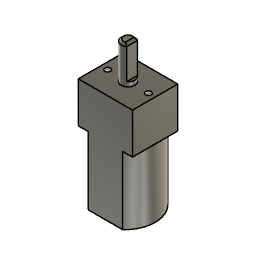
Gripper-3dita v34 (Autodesk Fusion 360 archive; units mm, degrees)
design "motore N20 A2.60RPM"
Autodesk Fusion 360 part; units mm, degrees
sketch "Schizzo1" plane through (0, 0, 0) normal (0, 0, 1) x (1, 0, 0)
  line L0 (-14.6061, 11.2687) -> (-2.6061, 11.2687) construction
  line L1 (-2.6061, 11.2687) -> (-2.6061, 1.2687)
  line L2 (-2.6061, 1.2687) -> (-14.6061, 1.2687) construction
  line L3 (-14.6061, 1.2687) -> (-14.6061, 11.2687)
  line L4 (-12.4061, 11.2687) -> (-4.8061, 11.2687)
  line L5 (-12.4061, 1.2687) -> (-4.8061, 1.2687)
  arc A0 (-12.4061, 11.2687) -> (-12.4061, 1.2687) centre (-7.8242, 6.2687) ccw
  arc A1 (-4.8061, 1.2687) -> (-4.8061, 11.2687) centre (-9.3879, 6.2687) ccw
  line L6 (-14.6061, 11.2687) -> (-2.6061, 1.2687)
  line L7 (-2.6061, 11.2687) -> (-14.6061, 1.2687)
  line L8 (-22.6061, 6.2687) -> (5.3939, 6.2687)
  dimension "d1" = 10
  dimension "d2" = 12
  dimension "d5" = 7.6
  dimension "d6" = 7.6
  constraint horizontal L0
  constraint vertical L1
  constraint horizontal L2
  constraint vertical L3
  constraint coincident L0 L4.start
  constraint parallel L0 L4
  constraint coincident L2 L5.start
  constraint parallel L2 L5
  constraint equal A0 A1
  constraint tangent L3 A0
  constraint tangent L1 A1
  constraint horizontal L8
  constraint midpoint L7 L8
  constraint coincident A1.centre L8
  measures "d1" distance of L0.start L2.end
  measures "d2" distance of L0.start L0.end
  measures "d5" distance of L4.start L4.end
  measures "d6" distance of L5.start L5.end
extrude "Estrusione1" add sketch "Schizzo1" along normal blind 15 contours A1 L7 L8 | A1 L6 L8 | L4 A0 A1 L6 L7 | L5 A0 A1 L6 L7 | A0 L6 L8 | A0 L7 L8
sketch "Schizzo2" plane through (0, 0, 15) normal (0, 0, 1) x (-1, 0, 0)
  arc A0 (12.4061, -11.2687) -> (12.4061, -1.2687) centre (7.8242, -6.2687) ccw
  line L0 (12.4061, -1.2687) -> (4.8061, -1.2687)
  arc A1 (4.8061, -1.2687) -> (4.8061, -11.2687) centre (9.3879, -6.2687) ccw
  line L1 (4.8061, -11.2687) -> (12.4061, -11.2687)
  line L2 (14.6061, -11.2687) -> (2.6061, -11.2687)
  line L3 (2.6061, -11.2687) -> (2.6061, -1.2687)
  line L4 (2.6061, -1.2687) -> (14.6061, -1.2687)
  line L5 (14.6061, -1.2687) -> (14.6061, -11.2687)
  constraint horizontal L2
  constraint vertical L3
  constraint horizontal L4
  constraint vertical L5
  constraint collinear L0 L4
  constraint collinear L1 L2
  constraint tangent A1 L3
  constraint tangent A0 L5
extrude "Estrusione2" add sketch "Schizzo2" along normal blind 9
sketch "Schizzo3" plane through (0, 0, 24) normal (0, 0, 1) x (-1, 0, 0)
  line L0 (14.6061, -1.2687) -> (2.6061, -1.2687)
  line L1 (2.6061, -1.2687) -> (2.6061, -11.2687)
  line L2 (2.6061, -11.2687) -> (14.6061, -11.2687)
  line L3 (14.6061, -11.2687) -> (14.6061, -1.2687)
  line L4 (8.6061, -1.2687) -> (8.6061, -11.2687)
  circle A0 centre (8.6061, -6.2687) radius 1.5
  dimension "d9" = 3
  constraint midpoint L0 L4.start
  constraint midpoint L2 L4.end
  constraint midpoint L4 A0.centre
  measures "d9" diameter of A0
extrude "Estrusione3" add sketch "Schizzo3" along normal blind 1 contours L4 A0 | L4 A0
sketch "Schizzo4" plane through (0, 0, 25) normal (0, 0, 1) x (-1, 0, 0)
  circle A0 centre (8.6061, -6.2687) radius 1.5
  line L0 (7.7061, -7.4687) -> (7.7061, -3.5)
  line L1 (7.7061, -3.5) -> (10.1061, -3.5)
  line L2 (10.1061, -3.5) -> (10.1061, -6.2687)
  arc A1 (7.7061, -7.4687) -> (7.7061, -5.0687) centre (8.6061, -6.2687) ccw
  dimension "d12" = 3
  dimension "d13" = 2.4
  constraint concentric A0 A1
  constraint vertical L0
  constraint horizontal L1
  constraint vertical L2
  constraint tangent L2 A1
  constraint coincident A0 L2.end
  constraint coincident A0 L0.start
  constraint coincident L0 A1.end
  measures "d12" diameter of A1
  measures "d13" distance of L0.end L1.end
extrude "Estrusione4" add sketch "Schizzo4" along normal blind 7.2 contours A0 L0 A1
chamfer "Smusso1" distance 0.5 angle 45 1 faces at (-8.4844, 6.1233, 32.2)
sketch "Schizzo5" plane through (0, 0, 0) normal (0, 0, -1) x (1, 0, 0)
  arc A0 (-12.4061, -1.2687) -> (-12.4061, -11.2687) centre (-7.8242, -6.2687) ccw
  line L0 (-12.4061, -11.2687) -> (-4.8061, -11.2687)
  arc A1 (-4.8061, -11.2687) -> (-4.8061, -1.2687) centre (-9.3879, -6.2687) ccw
  line L1 (-4.8061, -1.2687) -> (-12.4061, -1.2687)
  circle A2 centre (-12.3093, -6.2383) radius 1.5561
  circle A3 centre (-5.3753, -6.1228) radius 1.5561
  constraint equal A2 A3
extrude "Estrusione5" add sketch "Schizzo5" along normal blind 2.039 contours A2 | A3
fillet "Raccordo1" radius 1.5 2 faces at (-12.7379, 6.5305, -2.039) (-4.8514, 6.3478, -2.039)
sketch "Schizzo6" plane through (0, 0, 24) normal (0, 0, 1) x (-1, 0, 0)
  circle A0 centre (8.6061, -6.2687) radius 1.5
  line L0 (14.6061, -1.2687) -> (2.6061, -1.2687)
  line L1 (2.6061, -1.2687) -> (2.6061, -11.2687)
  line L2 (2.6061, -11.2687) -> (14.6061, -11.2687)
  line L3 (14.6061, -11.2687) -> (14.6061, -1.2687)
  line L4 (13.1061, -6.2687) -> (4.1061, -6.2687)
  point P0 (13.1061, -6.2687)
  point P1 (4.1061, -6.2687)
  dimension "d21" = 9
  constraint perpendicular L3 L4
  constraint midpoint A0.centre L4
  constraint coincident P0 L4.start
  constraint coincident P1 L4.end
  measures "d21" distance of P0 P1
hole "Foratura1" at (-13.1061, 6.2687, 24) at (-4.1061, 6.2687, 24) direction (0, 0, -1) diameter 1.271 depth 6 tip angle 118
thread "Filettatura1" "ISO Metric profile 1.6 M1.6x0.35 6H" thread offset 0 thread depth 7.4

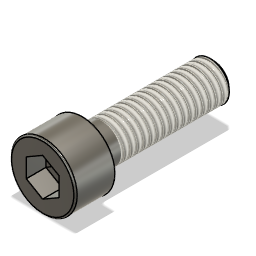
design "Vite a testa incassata JIS B 1176 - M6 x 1 x 20 Acciaio 4.6 Radente"
description: Vite a testa incassata JIS B 1176 - M6 x 1 x 20
part number: JIS B 1176 - M6 x 1 x 20 Acciaio 4.6 Radente
Autodesk Fusion 360 part; units mm, degrees
sketch "Sketch1" plane through (0, 0, 0) normal (0, 1, 0) x (1, 0, 0)
  line L0 (-3, 0) -> (-3, 20)
  line L1 (-3, 20) -> (0, 20)
  line L2 (0, 20) -> (0, -6)
  line L3 (-3, 0) -> (-5, 0)
  line L4 (-5, 0) -> (-5, -6)
  line L5 (-5, -6) -> (0, -6)
  dimension "d9" = 6
  dimension "d66" = 10
  dimension "d108" = 20
  dimension "d109" = 6
  constraint perpendicular L0 L1
  constraint collinear origin L1.end L2.end
  constraint perpendicular L0 L3
  constraint coincident origin L3
  constraint vertical L0
  constraint vertical L2
  constraint parallel L2 L4
  constraint coincident L2 L5.end
  constraint perpendicular L2 L5
  measures "d108" distance of origin L1
  measures "d109" distance of L3.end L5
revolve "Revolve1" add sketch "Sketch1" angle 360 about axis through (0, 0, -20) along (0, 0, 1)
ref_plane "WorkPlane1" through (0, 0, 6) normal (0, 0, 1) x (1, 0, 0)
sketch "Sketch6" plane through (0, 0, 6) normal (0, 0, 1) x (1, 0, 0)
  line L0 (-2.5, 0) -> (2.5, 0) construction
  line L1 (0, 0) -> (-2.5, 1.4434)
  line L2 (-2.5, -1.4434) -> (-2.5, 1.4434)
  line L3 (-2.5, -1.4434) -> (0, 0)
  dimension "d97" = 150
  dimension "d110" = 5
  constraint horizontal L0
  constraint midpoint L1.start L0
  constraint coincident L1.start L3.end
  constraint perpendicular L0 L2
  constraint midpoint L0.start L2
  constraint coincident L1.end L2.end
  measures "d97" angle of L0 L1
  measures "d110" distance of L0.end L2
extrude "Extrude1" cut sketch "Sketch6" against normal blind 3
pattern_circular "C-Pattern1" count 6 over 360 about axis through (0, 0, 1.75) along (0, 0, 1) of "Extrude1"
extrude "Extrude2" cut 1 faces at (0.8333, -0.4811, 3) along direction (0, 0, -1) blind 3 draft -85
thread "Thread2" "ISO Metric profile 6.0 M6x1 6g" major diameter 5.884 minor diameter 4.7435 pitch 1 angle 60 resizes the face on face at (-2.9851, 0.2987, -13.3333) from (0, 0, -3) to (0, 0, -20)
sketch "Sketch7" plane through (0, 0, 0) normal (0, 1, 0) x (1, 0, 0)
  line L0 (-3.06, 20) -> (-3.06, 19.3865)
  line L1 (-3.06, 19.3865) -> (-2.3865, 20)
  line L2 (0, 20) -> (0, -6)
  line L3 (-3.06, 20) -> (0, 20)
  dimension "d111" = 2.3866
  dimension "d112" = 3.06
  dimension "d113" = 0.6135
  constraint coincident L2.start L3.end
  constraint perpendicular L0 L3
  constraint coincident L1.end L3
  constraint perpendicular L2 L3
  measures "d111" distance of L1.end L2
  measures "d112" distance of L0 L2.start
  measures "d113" distance of L0.end L3
revolve "Revolve3" cut sketch "Sketch7" angle 360 about axis through (0, 0, 1.75) along (0, 0, 1)
fillet "Fillet5" radius 0.25 1 edges at (-4.6616, 1.8081, 6)
fillet "Fillet7" radius 0.6 1 edges at (2.7429, -1.0639, 0)
equation "d9 = adsk_nomdia"
equation "adsk_nomlen = 20.00 mm"
equation "adsk_headh = 6.00 mm"
equation "adsk_headdia = 10.00 mm"
equation "adsk_nomdia = 6.00 mm"
equation "adsk_philwidth = 5.00 mm"
equation "d31 = -adsk_phildepth"
equation "adsk_phildepth = 3.00 mm"
equation "d66 = adsk_headdia"
equation "d71 = adsk_headh"
equation "d76 = -adsk_phildepth"
equation "adsk_thrlen = 17.00 mm"
equation "d84 = adsk_thrlen"
equation "adsk_startlen = 0.61345 mm"
equation "adsk_endpointdia = 4.7731 mm"
equation "adsk_headtoprad = 0.25 mm"
equation "d102 = adsk_headtoprad"
equation "adsk_midfillet = 0.60 mm"
equation "d107 = adsk_midfillet"
equation "d108 = adsk_nomlen"
equation "d109 = adsk_headh"
equation "d110 = adsk_philwidth"
equation "d111 = adsk_endpointdia / 2"
equation "d112 = adsk_nomdia * 0.51"
equation "d113 = adsk_startlen"

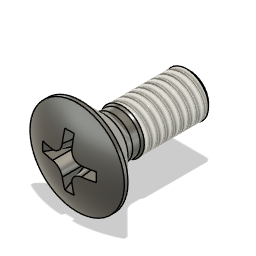
design "Vite a testa rialzata svasata UNI EN ISO 7047 - M4 x 10 - H Acciaio 4.6 Radente"
description: Vite a testa rialzata svasata UNI EN ISO 7047 - M4 x 10 - H
part number: UNI EN ISO 7047 - M4x10 - H Acciaio 4.6 Radente
Autodesk Fusion 360 part; units mm, degrees
sketch "Sketch1" plane through (0, 0, 0) normal (0, 1, 0) x (1, 0, 0)
  line L0 (-4.2, -4.525) -> (-4.2, -4.2)
  line L1 (-4.2, -4.2) -> (-1.825, -1.825)
  line L2 (-2, 5.475) -> (0, 5.475)
  line L3 (0, 5.475) -> (0, -5.525)
  arc A0 (-4.2, -4.525) -> (0, -5.525) centre (0, 3.795) ccw
  line L4 (-1.825, -1.825) -> (-1.825, -0.7281)
  line L5 (-2, -0.425) -> (-2, 5.475)
  line L6 (-2, -0.425) -> (-1.825, -0.7281)
  dimension "d9" = 4
  dimension "d11" = 8.4
  dimension "d68" = 10
  dimension "d90" = 2.7
  dimension "d91" = 1
  dimension "d93" = 3.65
  dimension "d135" = 5.9
  dimension "d157" = 45
  dimension "d160" = 30
  constraint vertical L0
  constraint vertical L3
  constraint coincident L3.end A0
  constraint coincident L3 A0.centre
  constraint vertical L4
  constraint parallel L4 L5
  constraint horizontal L2
  constraint coincident origin L3
  constraint coincident origin L1
  measures "d68" vertical distance of L0.start L2.start
  measures "d90" vertical distance of L0.start L1.end
  measures "d91" vertical distance of L3.end L0.start
  measures "d135" distance of L2 L5.start
  measures "d157" angle of L1 L3
  measures "d160" angle of L5 L6
revolve "Revolve1" add sketch "Sketch1" angle 360 about axis through (0, 0, -5.475) along (0, 0, 1) makes body 1
ref_plane "WorkPlane1" through (0, 0, 5.525) normal (0, 0, 1) x (1, 0, 0)
sketch "Sketch2" plane through (0, 0, 5.525) normal (0, 0, 1) x (1, 0, 0)
  line L0 (-0.4333, 2.6) -> (-0.4333, 0.4333)
  line L1 (-0.4333, 0.4333) -> (-2.6, 0.4333)
  line L2 (0, 0) -> (0, 2.6) construction
  line L3 (-0.4333, 2.6) -> (0.4333, 2.6)
  line L4 (-2.6, 0.4333) -> (-2.6, -0.4333)
  circle A0 centre (0, 0) radius 4.2
  line L5 (0, 0) -> (-4.2, 0) construction
  line L6 (2.6, 0.4333) -> (2.6, -0.4333)
  line L7 (0.4333, 0.4333) -> (2.6, 0.4333)
  line L8 (0.4333, 2.6) -> (0.4333, 0.4333)
  line L9 (-0.4333, -0.4333) -> (-2.6, -0.4333)
  line L10 (-0.4333, -2.6) -> (-0.4333, -0.4333)
  line L11 (-0.4333, -2.6) -> (0.4333, -2.6)
  line L12 (0.4333, -2.6) -> (0.4333, -0.4333)
  line L13 (0.4333, -0.4333) -> (2.6, -0.4333)
  dimension "d22" = 0.8667
  dimension "d161" = 5.2
  constraint perpendicular L0 L1
  constraint equal L3 L4
  constraint equal L0 L1
  constraint horizontal L0.start L2.end
  constraint vertical L2
  constraint coincident L2.start A0.centre
  constraint perpendicular L4 L5
  constraint coincident A0 L5.end
  constraint horizontal L5
  constraint vertical L0
  constraint symmetric L0.start L2 L3.end
  constraint symmetric L0.end L2 L7.start
  constraint symmetric L1.end L2 L6.start
  constraint symmetric L2 L4.end L6.end
  constraint coincident L3.end L8.start
  constraint symmetric L0.start L5 L10.start
  constraint symmetric L0.end L5 L9.start
  constraint symmetric L1.end L5 L4.end
  constraint symmetric L3.end L5 L11.end
  constraint symmetric L5 L6.start L6.end
  constraint symmetric L5 L7.start L12.end
  constraint symmetric L5 L3.end L11.end
  constraint coincident L6.end L13.end
  measures "d22" horizontal distance of L0.start L3.end
  measures "d161" distance of L1.end L6.start
extrude "Extrude1" add sketch "Sketch2" against normal blind 3.2 draft -4 separate body contours L0 L1 L3 L4 L6 L7 L8 L9 L10 L11 L12 L13 makes body 2
draft "Draft1" angle -30 neutral plane through (0, 0, 5.525) pull (0, 0, 1) 4 faces at (-2.5254, 0.0699, 4.4583) (0.0699, 2.5254, 4.4583) (0.0699, -2.5254, 4.4583) (2.5254, 0.0699, 4.4583) on bodies 2
fillet "Fillet3" radius 0.8667 4 edges at (-0.3215, 0.3215, 3.925) (0.3215, 0.3215, 3.925) (0.3215, -0.3215, 3.925) (-0.3215, -0.3215, 3.925) on bodies 2
combine "Combine1" operation cut target body 1 tool bodies 2
fillet "Fillet7" radius 1 1 edges at (-1.7015, 0.6599, 1.825) on bodies 1
thread "Thread1" "ISO Metric profile 4.0 M4x0.7 6g" major diameter 3.908 minor diameter 3.111 pitch 0.7 angle 60 resizes the face on face at (-1.9975, 0.0997, -1.5417) on bodies 1
sketch "Sketch7" plane through (0, 0, 0) normal (0, 1, 0) x (1, 0, 0)
  line L0 (-1.69, 5.475) -> (-2.04, 5.475)
  line L1 (-2.04, 5.475) -> (-2.04, 5.125)
  line L2 (-2.04, 5.125) -> (-1.69, 5.475)
  point P0 (0, 5.475)
  dimension "d152" = 45
  dimension "d154" = 0.35
  dimension "d155" = 2.04
  constraint horizontal L0
  constraint perpendicular L0 L1
  constraint coincident L0 P0
  measures "d152" angle of L1 L2
  measures "d154" distance of L0.end L1.end
  measures "d155" distance of L1 P0
revolve "Revolve3" cut sketch "Sketch7" angle 360 about axis through (0, 0, 1.75) along (0, 0, 1) bodies 1
equation "d9 = adsk_nomdia"
equation "d11 = adsk_headdia"
equation "d22 = adsk_philwidth"
equation "d31 = -adsk_phildepth"
equation "d59 = adsk_philwidth"
equation "d68 = adsk_nomlen"
equation "d71 = adsk_shnkdia * 0.5 / tan(adsk_headang * 0.5) + adsk_headh + adsk_ovalh"
equation "d90 = adsk_headh"
equation "d91 = adsk_ovalh"
equation "d93 = adsk_shnkdia"
equation "adsk_headang = 90.00 deg"
equation "adsk_nomlen = 10.00 mm"
equation "adsk_headh = 2.70 mm"
equation "adsk_headdia = 8.40 mm"
equation "adsk_nomdia = 4.00 mm"
equation "adsk_phildia = 5.20 mm"
equation "adsk_philwidth = adsk_phildia / 6"
equation "adsk_phildepth = 3.20 mm"
equation "adsk_ovalh = 1.00 mm"
equation "adsk_thrlen = 5.90 mm"
equation "adsk_shnkdia = adsk_nomdia - 0.5 * adsk_pitch1"
equation "d135 = adsk_thrlen"
equation "adsk_pitch1 = 0.70 mm"
equation "adsk_midfillet = 1.00 mm"
equation "d143 = adsk_midfillet"
equation "d150 = ( adsk_shnkdia * 0.5 ) * tan(90 deg - adsk_headang * 0.5) + adsk_headh"
equation "d154 = adsk_pitch1 * 0.5"
equation "d155 = adsk_nomdia * 0.51"
equation "d161 = adsk_phildia"

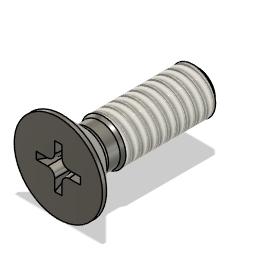
design "Vite a testa piatta svasata UNI EN ISO 7046-1 - M2 x 6 - H Acciaio 4.6 Radente"
description: Vite a testa piatta svasata UNI EN ISO 7046-1 - M2 x 6 - H
part number: UNI EN ISO 7046-1 - M2 x 6 - H Acciaio 4.6 Radente
Autodesk Fusion 360 part; units mm, degrees
sketch "Sketch1" plane through (0, 0, 0) normal (0, 1, 0) x (1, 0, 0)
  line L0 (0, -2.0773) -> (-1.9, -2.0773)
  line L1 (-1.9, -2.0773) -> (-1.9, -1.9)
  line L2 (-1.9, -1.9) -> (-0.8773, -0.8773)
  line L3 (-1, -0.0773) -> (-1, 3.9227)
  line L4 (-0.8773, -0.8773) -> (0, 0) construction
  line L5 (-1, 3.9227) -> (0, 3.9227)
  line L6 (0, 3.9227) -> (0, -2.0773)
  line L7 (-0.8773, -0.2898) -> (-0.8773, -0.8773)
  line L8 (-1, -0.0773) -> (-0.8773, -0.2898)
  dimension "d5" = 45
  dimension "d9" = 2
  dimension "d11" = 3.8
  dimension "d71" = 1.2
  dimension "d72" = 1.7546
  dimension "d89" = 4
  dimension "d101" = 30
  dimension "d115" = 6
  constraint perpendicular L0 L1
  constraint vertical L3
  constraint perpendicular L3 L5
  constraint collinear L2 L4
  constraint perpendicular L0 L6
  constraint collinear L4.end L0.start L5.end
  constraint coincident L4.end L6
  constraint coincident origin L4
  constraint horizontal L0
  constraint coincident L2.end L4.start
  constraint coincident L7 L8.end
  constraint coincident L7.start L8.end
  measures "d5" angle of L4 L6
  measures "d71" distance of L0 L2.end
  measures "d89" distance of L5 L3.start
  measures "d101" angle of L3 L8
  measures "d115" distance of L0.start L5
revolve "Revolve1" add sketch "Sketch1" angle 360 about axis through (0, 0, -3.9227) along (0, 0, 1) makes body 1
sketch "Sketch2" plane through (0, 0, 2.0773) normal (0, 0, 1) x (1, 0, 0)
  line L0 (-0.155, 0.155) -> (-0.95, 0.155)
  line L1 (-0.95, 0.155) -> (-0.95, -0.155)
  line L2 (-0.95, -0.155) -> (-0.155, -0.155)
  line L3 (0.155, -0.95) -> (0.155, -0.155)
  line L4 (-0.155, -0.95) -> (0.155, -0.95)
  line L5 (-0.155, -0.155) -> (-0.155, -0.95)
  line L6 (0.95, 0.155) -> (0.155, 0.155)
  line L7 (0.95, -0.155) -> (0.95, 0.155)
  line L8 (0.155, -0.155) -> (0.95, -0.155)
  line L9 (-0.155, 0.95) -> (-0.155, 0.155)
  line L10 (0.155, 0.95) -> (-0.155, 0.95)
  line L11 (0.155, 0.155) -> (0.155, 0.95)
  dimension "d111" = 360
  dimension "d116" = 0.31
  dimension "d117" = 1.9
  constraint horizontal L0
  constraint perpendicular L0 L1
  constraint horizontal L2
  constraint vertical L0.start L2.end
  constraint coincident L0.start L9.end
  measures "d116" distance of L0 L1.end
  measures "d117" distance of L4.start L10
extrude "Extrude1" add sketch "Sketch2" against normal blind 1.2 draft -4 separate body makes body 2
draft "Draft1" angle -30 neutral plane through (0, 0, 2.0773) pull (0, 0, 1) 4 faces at (0.922, 0.0237, 1.6773) (-0.0237, 0.922, 1.6773) (-0.922, -0.0237, 1.6773) (0.0237, -0.922, 1.6773) on bodies 2
fillet "Fillet3" radius 0.31 4 edges at (0.113, 0.113, 1.4773) (0.113, -0.113, 1.4773) (-0.113, -0.113, 1.4773) (-0.113, 0.113, 1.4773) on bodies 2
combine "Combine1" operation cut target body 1 tool bodies 2
thread "Thread1" "ISO Metric profile 2.0 M2x0.4 6g" major diameter 1.9335 minor diameter 1.478 pitch 0.4 angle 60 resizes the face on face at (-0.9988, 0.0498, -1.256) on bodies 1
fillet "Fillet5" radius 0.2 1 edges at (-0.8179, 0.3172, 0.8773) on bodies 1
sketch "Sketch6" plane through (0, 0, 0) normal (0, 1, 0) x (1, 0, 0)
  line L0 (-0.7546, 3.9227) -> (-1.02, 3.9227)
  line L1 (-1.02, 3.9227) -> (-1.02, 3.6773)
  line L2 (-1.02, 3.6773) -> (-0.7546, 3.9227)
  line L3 (-1, 3.9227) -> (0, 3.9227)
  line L4 (0, 0) -> (0, 3.9227) construction
  dimension "d102" = 1.02
  dimension "d118" = 0.7546
  dimension "d119" = 0.2454
  constraint horizontal L0
  constraint perpendicular L0 L1
  constraint coincident L0.start L3
  constraint coincident L4.start origin
  constraint coincident L3.end L4.end
  measures "d102" distance of L4.start L1
  measures "d118" distance of L0.start L4
  measures "d119" distance of L0 L1.end
revolve "Revolve3" cut sketch "Sketch6" angle 360 about axis through (0, 0, 1.75) along (0, 0, 1) bodies 1
equation "d5 = adsk_headang * 0.5"
equation "d9 = adsk_nomdia"
equation "d11 = adsk_headdia"
equation "adsk_nomlen = 6.00 mm"
equation "adsk_headh = 1.20 mm"
equation "adsk_headdia = 3.80 mm"
equation "adsk_nomdia = 2.00 mm"
equation "adsk_headang = 90.00 deg"
equation "adsk_phildia = 1.90 mm"
equation "d31 = -adsk_phildepth"
equation "adsk_philwidth = 0.31 mm"
equation "adsk_phildepth = 1.20 mm"
equation "d71 = adsk_headh"
equation "d72 = adsk_shnkdia"
equation "adsk_shnkdia = 1.75462 mm"
equation "d89 = adsk_thrlen"
equation "adsk_thrlen = 4.00 mm"
equation "adsk_pitch1 = 0.40 mm"
equation "adsk_startlen = 0.24538 mm"
equation "adsk_midfillet = adsk_nomdia * 0.1"
equation "d96 = adsk_midfillet"
equation "d99 = ( adsk_shnkdia / 2 ) * tan(90 deg - adsk_headang / 2) + adsk_headh"
equation "d102 = adsk_nomdia * 0.51"
equation "adsk_endpointdia = 1.50924 mm"
equation "d114 = adsk_philwidth"
equation "d115 = adsk_nomlen"
equation "d116 = adsk_philwidth"
equation "d117 = adsk_phildia"
equation "d118 = adsk_endpointdia / 2"
equation "d119 = adsk_startlen"

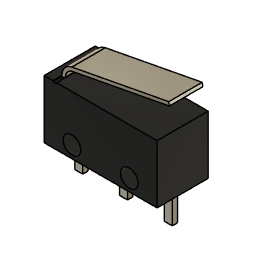
design "microswitch"
Autodesk Fusion 360 part; units mm, degrees
sketch "Schizzo1" plane through (0, 0, 0) normal (0, 1, 0) x (1, 0, 0)
  line L0 (0, 0) -> (12.8, 0)
  line L1 (12.8, 0) -> (12.8, -6.6)
  line L2 (12.8, -6.6) -> (0, -6.6)
  line L3 (0, -6.6) -> (0, 0)
  circle A0 centre (3.15, -1.35) radius 1
  circle A1 centre (9.65, -1.35) radius 1
  line L4 (0, -1.35) -> (3.15, -1.35) construction
  line L5 (3.15, -1.35) -> (9.65, -1.35) construction
  line L6 (9.65, -1.35) -> (12.8, -1.35) construction
  line L7 (1, -6.6) -> (1, -6.5)
  line L8 (1, -6.5) -> (1.4, -6.5)
  line L9 (1.4, -6.5) -> (1.4, -6.6)
  dimension "d1" = 6.6
  dimension "d2" = 12.8
  dimension "d3" = 2
  dimension "d4" = 2
  dimension "d5" = 6.5
  dimension "d6" = 5.25
  dimension "d7" = 1
  dimension "d8" = 0.1
  dimension "d9" = 0.4
  dimension "d28" = 6.6
  constraint horizontal L0
  constraint vertical L1
  constraint horizontal L2
  constraint vertical L3
  constraint coincident L0.start L3.end
  constraint coincident L3 L4.start
  constraint coincident A0.centre L4.end
  constraint perpendicular L3 L4
  constraint coincident A1.centre L5.end
  constraint coincident L1 L6.end
  constraint perpendicular L1 L6
  constraint horizontal L5
  constraint equal L4 L6
  constraint coincident L2 L7.start
  constraint perpendicular L2 L7
  constraint perpendicular L7 L8
  constraint coincident L2 L9.end
  constraint perpendicular L2 L9
  measures "d1" distance of L0.start L2.end
  measures "d2" distance of L0.start L0.end
  measures "d3" diameter of A0
  measures "d4" diameter of A1
  measures "d5" distance of A0.centre A1.centre
  measures "d6" distance of L2 L5
  measures "d7" distance of L3 L7
  measures "d8" distance of L7.start L7.end
  measures "d9" distance of L7.end L8.end
  measures "d28" distance of L0.end L1.end
extrude "Estrusione1" add sketch "Schizzo1" along normal mid plane 5.8 contours L0 L1 L2 L3 L7 L8 L9 makes body 1
sketch "Schizzo2" plane through (0, 0, 0) normal (0, 1, 0) x (1, 0, 0)
  arc A0 (1.4, -6.6275) -> (2.2125, -7.6097) centre (2.4, -6.6275) ccw
  line L0 (2.2125, -7.6097) -> (13.2, -9.7071)
  line L1 (0, -6.6) -> (0, 0)
  line L2 (0, 0) -> (12.8, 0)
  arc A1 (1, -6.6275) -> (2.1375, -8.0026) centre (2.4, -6.6275) ccw
  line L3 (2.1375, -8.0026) -> (13.125, -10.1)
  line L4 (13.125, -10.1) -> (13.2, -9.7071)
  circle A2 centre (9.65, -1.35) radius 1
  line L5 (1, -6.6275) -> (1, -6.5)
  line L6 (1, -6.5) -> (1.4, -6.5)
  line L7 (1.4, -6.5) -> (1.4, -6.6275)
  line L8 (1, -6.5) -> (1, -6.6)
  line L9 (1.4, -6.5) -> (1, -6.5)
  line L10 (1.4, -6.6) -> (1.4, -6.5)
  point P0 (13.1818, -7.4)
  dimension "d13" = 1
  dimension "d14" = 13.2
  dimension "d16" = 0.4
  dimension "d17" = 10.1
  dimension "d29" = 3.475
  dimension "d30" = 7.4
  constraint tangent A0 L0
  constraint perpendicular L0 L4
  constraint vertical L5
  constraint perpendicular L5 L6
  constraint perpendicular L6 L7
  constraint collinear L5 L8
  constraint collinear L6 L9
  constraint collinear L7 L10
  constraint tangent A1 L5
  constraint tangent A0 L7
  measures "d13" radius of A0
  measures "d14" distance of L0.end L1
  measures "d17" vertical distance of L2.end L3.end
  measures "d29" horizontal distance of L3.end A2.centre
  measures "d30" vertical distance of L2.end P0
extrude "Estrusione2" add sketch "Schizzo2" along normal mid plane 3.8 separate body contours A0 L0 A1 L3 L4 L5 L6 L7 L8 L9 L10 makes body 2
sketch "Schizzo3" plane through (0, 0, 0) normal (0, 0, -1) x (1, 0, 0)
  line L0 (0, 2.9) -> (0, -2.9)
  line L1 (0, -2.9) -> (12.8, -2.9)
  line L2 (12.8, -2.9) -> (12.8, 2.9)
  line L3 (12.8, 2.9) -> (0, 2.9)
  line L4 (5.95, 0.3) -> (6.85, 0.3)
  line L5 (6.85, 0.3) -> (6.85, -0.3)
  line L6 (6.85, -0.3) -> (5.95, -0.3)
  line L7 (5.95, -0.3) -> (5.95, 0.3)
  line L8 (5.95, 0) -> (6.85, 0) construction
  line L9 (6.4, 2.9) -> (6.4, -2.9) construction
  line L10 (0.87, -0.3) -> (0.87, 0.3)
  line L11 (0.87, 0.3) -> (1.77, 0.3)
  line L12 (0.87, 0) -> (1.77, 0) construction
  line L13 (1.77, -0.3) -> (0.87, -0.3)
  line L14 (1.77, 0.3) -> (1.77, -0.3)
  line L15 (11.03, -0.3) -> (11.03, 0.3)
  line L16 (11.03, 0.3) -> (11.93, 0.3)
  line L17 (11.03, 0) -> (11.93, 0) construction
  line L18 (11.93, -0.3) -> (11.03, -0.3)
  line L19 (11.93, 0.3) -> (11.93, -0.3)
  dimension "d20" = 0.9
  dimension "d21" = 0.6
  dimension "d24" = 5.08
  dimension "d25" = 0
  constraint horizontal L4
  constraint vertical L5
  constraint horizontal L6
  constraint vertical L7
  constraint midpoint L7 L8.start
  constraint midpoint L5 L8.end
  constraint midpoint L3 L9.start
  constraint midpoint L1 L9.end
  constraint midpoint L8 L9
  measures "d20" distance of L4.start L4.end
  measures "d21" distance of L4.start L6.end
extrude "Estrusione3" add sketch "Schizzo3" along normal blind 3.5 separate body contours L4 L5 L6 L7 | L10 L11 L13 L14 | L15 L16 L18 L19 makes body 3 at (1.17, -0.3, -1.1667) makes body 4 at (6.25, -0.3, -1.1667) makes body 5 at (11.33, -0.3, -1.1667)
copy_body "Corpo->Comp1" bodies 1 removing the originals makes body 6 in component "Component"
copy_body "Corpo->Comp2" bodies 2 removing the originals makes body 7 in component "Component'"
copy_body "Corpo->Comp3" bodies 3 removing the originals makes body 8 in component "Component''"
copy_body "Corpo->Comp4" bodies 4 removing the originals makes body 9 in component "Component'''"
copy_body "Corpo->Comp5" bodies 5 removing the originals makes body 10 in component "Component''''"
component "Component" placed x (1, 0, 0) y (0, 1, 0) z (0, 0, 1) at (0, 0, 0)
component "Component'" placed x (1, 0, 0) y (0, 1, 0) z (0, 0, 1) at (0, 0, 0)
component "Component''" placed x (1, 0, 0) y (0, 1, 0) z (0, 0, 1) at (0, 0, 0)
component "Component'''" placed x (1, 0, 0) y (0, 1, 0) z (0, 0, 1) at (0, 0, 0)
component "Component''''" placed x (1, 0, 0) y (0, 1, 0) z (0, 0, 1) at (0, 0, 0)
equation "d6 = 6.6 mm - 0.35 mm - 1 mm"
